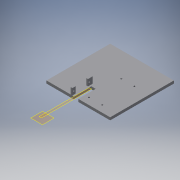
# Autodesk Inventor part: MainBoard
Saved by Autodesk Inventor 2018 (Build 220112000, 112)
## iProperties
Created: 2018-09-19
Part Number: MainBoard
Material: Generic
Document SubType Name: Modeling
Designer: Viraj Shah
Mass: 47.0321 g
Surface Area: 216.401 cm^2
Volume: 47.0321 cm^3
Density: 1 g/cm^3
Appearance: Default
Author: Viraj Shah
Autodesk Inventor part; units mm, degrees
ref_plane "YZ Plane" through (0, 0, 0) normal (1, 0, 0) x (0, 1, 0)
ref_plane "XZ Plane" through (0, 0, 0) normal (0, 1, 0) x (-1, 0, 0)
ref_plane "XY Plane" through (0, 0, 0) normal (0, 0, 1) x (1, 0, 0)
ref_plane "Work Plane1" through (0, 0, -6.5) normal (0, 0, 1) x (1, 0, 0)
ref_plane "Work Plane4" through (0, 0, -7.75) normal (0, 0, 1) x (1, 0, 0)
sketch "Sketch3" plane through (0, 0, -7.75) normal (0, 0, 1) x (1, 0, 0)
  line L0 (42.5701, 64.9855) -> (2.5701, 64.9855) projected
  line L1 (2.5701, 97.7078) -> (2.5701, 64.9855)
  line L2 (2.5701, 64.9855) -> (42.5701, 64.9855)
  line L3 (42.5701, 184.9855) -> (-37.4299, 184.9855)
  line L4 (-5.7403, 64.9855) -> (-37.4299, 64.9855)
  line L5 (-5.7403, 64.9855) -> (-5.7403, 97.7078)
  line L6 (-5.7403, 97.7078) -> (2.5701, 97.7078)
  line L7 (-37.4299, 64.9855) -> (-57.4299, 64.9855)
  line L8 (-57.4299, 64.9855) -> (-57.4299, 184.9855)
  line L9 (-37.4299, 184.9855) -> (-57.4299, 184.9855)
  line L10 (42.5701, 64.9855) -> (62.5701, 64.9855)
  line L11 (62.5701, 64.9855) -> (62.5701, 184.9855)
  line L12 (42.5701, 184.9855) -> (62.5701, 184.9855)
  point P0 (0, 0)
  point P1 (-47.4299, 184.9855)
  dimension "d11" = 40
  dimension "d39" = 20
  dimension "d40" = 20
  constraints: 24 end point, 5 horizontal, 2 perpendicular, 2 vertical, 1 point on line
  measures "d11" distance of L0.start L0.end
  measures "d39" distance of L4.end L7.end
  measures "d40" distance of L0.start L10.end
extrude "Extrusion2" add sketch "Sketch3" against normal blind 5
sketch "Sketch4" plane through (0, 0, -7.75) normal (0, 0, 1) x (1, 0, 0)
  line L0 (-5.7403, 64.9855) -> (-57.4299, 64.9855) projected
  line L1 (-8.6817, 64.9855) -> (-11.6817, 64.9855)
  line L2 (-11.6817, 64.9855) -> (-11.6817, 70.9855)
  line L3 (-11.6817, 70.9855) -> (-8.6817, 70.9855)
  line L4 (-8.6817, 70.9855) -> (-8.6817, 64.9855)
  line L5 (-8.6817, 94.4855) -> (-11.6817, 94.4855)
  line L6 (-11.6817, 94.4855) -> (-11.6817, 103.4855)
  line L7 (-11.6817, 103.4855) -> (-8.6817, 103.4855)
  line L8 (-8.6817, 103.4855) -> (-8.6817, 94.4855)
  point P0 (0, 0)
  point P1 (-37.4299, 64.9855)
  dimension "d13" = 3
  dimension "d14" = 6
  dimension "d15" = 3
  dimension "d16" = 9
  dimension "d17" = 23.5
  constraints: 16 end point, 4 parallel, 2 horizontal, 2 perpendicular, 1 point on line
  measures "d13" distance of L2.end L3.end
  measures "d14" distance of L1.end L2.end
  measures "d15" distance of L6.end L7.end
  measures "d16" distance of L5.end L6.end
  measures "d17" distance between parallel lines of L3 L5
extrude "Extrusion3" add sketch "Sketch4" along normal blind 12
sketch "Sketch5" plane through (-8.6817, 64.9855, -7.75) normal (1, 0, 0) x (0, 0, -1)
  line L0 (0, 0) -> (0, 120) projected
  line L1 (0, 0) -> (-12, 0) projected
  point P0 (-7.75, -64.9855)
  point P1 (-6, 3)
  point P2 (-6, 32)
  dimension "d20" = 6
  dimension "d21" = 3
  dimension "d22" = 29
  measures "d20" distance from line of point (-6, 3) L0
  measures "d21" distance from line of L1 point (-6, 3)
  measures "d22" distance of point (-6, 32) point (-6, 3)
hole "Hole1" at (-8.6817, 67.9855, -1.75) at (-8.6817, 96.9855, -1.75) direction (-1, 0, 0) diameter 2.5 end through all
sketch "Sketch7" plane through (0, 0, -7.75) normal (0, 0, 1) x (1, 0, 0)
  circle A0 centre (30.2201, 77.6355) radius 1.375 projected
  circle A1 centre (30.2201, 138.3355) radius 1.375 projected
  circle A2 centre (54.9201, 138.3355) radius 1.375 projected
  circle A3 centre (54.9201, 77.6355) radius 1.375 projected
  point P0 (0, 0)
extrude "Extrusion4" cut sketch "Sketch7" against normal blind 12
body "Solid2"
